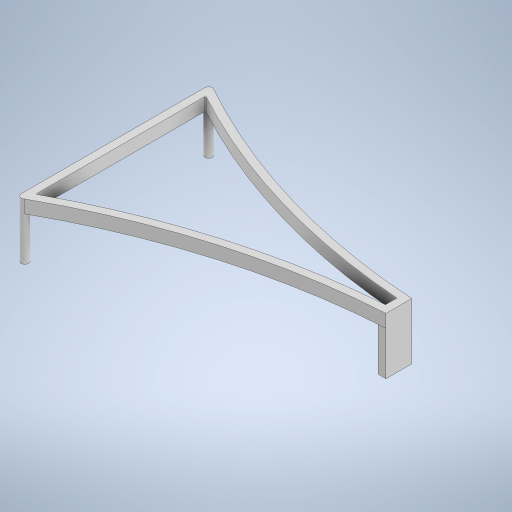
# Autodesk Inventor part: drzak_baterie
Saved by Autodesk Inventor 2024 (Build 280153000, 153)
## iProperties
Created: 2024-04-17
Part Number: drzak_baterie
Material: Všeobecné
Document SubType Name: Modeling
Designer: eliasla
Density: 1 g/cm^3
Appearance: Výchozí
Author: eliasla
Autodesk Inventor part; units mm, degrees
ref_plane "YZ Plane" through (0, 0, 0) normal (1, 0, 0) x (0, 1, 0)
ref_plane "XZ Plane" through (0, 0, 0) normal (0, 1, 0) x (-1, 0, 0)
ref_plane "XY Plane" through (0, 0, 0) normal (0, 0, 1) x (1, 0, 0)
sketch "Náčrt1" plane through (0, 0, 0) normal (0, 0, 1) x (1, 0, 0)
  line L0 (47.8317, -5) -> (50.8317, -5)
  line L1 (50.8317, -5) -> (50.8317, 5)
  line L2 (50.8317, 5) -> (47.8317, 5)
  line L3 (47.8317, 5) -> (47.8317, -5)
  line L4 (47.8317, -5) -> (50.8317, 5) construction
  line L5 (50.8317, -5) -> (47.8317, 5) construction
  circle A0 centre (-58.7223, 35.7005) radius 1.45
  circle A1 centre (-58.7223, -35.5995) radius 1.45
  point P0 (0, 0)
  point P1 (50.8317, 0)
  point P2 (-60.1683, 0.0505)
  dimension "d7" = 10
  dimension "d8" = 5
  dimension "d13" = 2.9
  dimension "d14" = 74.2
  constraints: 12 end point, 2 centre point, 2 parallel, 1 horizontal, 1 midpoint, 1 perpendicular
  measures "d7" distance of L0.end L1.end
  measures "d8" vertical distance of point (0, 0) L2.end
  measures "d13" diameter of A0
extrude "Vysunutí1" add sketch "Náčrt1" along normal blind 17
sketch "Náčrt2" plane through (-58.7223, 35.7005, 17) normal (0, 0, 1) x (1, 0, 0)
  circle A0 centre (0, 0) radius 1.45 projected
  line L0 (109.5541, -40.7005) -> (109.5541, -30.7005) projected
  arc A1 (0.9632, 1.0839) -> (109.5541, -30.7005) centre (125.5077, 225.1962) ccw
  circle A2 centre (0, -71.3) radius 1.45 projected
  line L1 (-1.45, 0) -> (-1.45, -71.3)
  arc A3 (109.5541, -40.7005) -> (0.9632, -72.3839) centre (125.3027, -296.61) ccw
  arc A4 (1.55, -3.0822) -> (1.9226, -2.8646) centre (0, 0) ccw
  line L2 (106.5541, -33.504) -> (106.5541, -37.8971)
  arc A5 (106.5541, -37.8971) -> (1.8423, -68.4842) centre (125.3027, -296.61) ccw
  arc A6 (1.8423, -68.4842) -> (1.55, -68.3189) centre (0, -71.4011) ccw
  line L3 (106.5541, -37.8971) -> (106.5541, -33.504)
  line L4 (1.55, -3.0822) -> (1.55, -68.3189)
  arc A7 (1.9226, -2.8646) -> (106.5541, -33.504) centre (125.5077, 225.1962) ccw
  line L5 (109.5541, -30.7005) -> (109.5541, -40.7005)
  arc A8 (0.4127, -72.69) -> (0.9632, -72.3839) centre (0, -71.3) ccw
  arc A9 (0.9632, 1.0839) -> (-1.45, 0) centre (0, 0) ccw
  arc A10 (0.9632, 1.0839) -> (-1.45, 0) centre (0, 0) ccw
  arc A11 (-1.45, -71.3) -> (0.9632, -72.3839) centre (0, -71.3) ccw
  point P0 (58.7223, -35.7005)
  point P1 (3.4391, -0.2742)
  point P2 (-1.45, -3.1305)
  point P3 (3.4391, -71.1268)
  point P4 (-1.45, -68.2706)
  point P5 (109.5541, -35.7005)
  point P6 (106.5541, -35.7005)
  dimension "d20" = 2
  dimension "d23" = 3
  constraints: 26 point on circle, 10 centre point, 10 end point, 4 coincident, 2 collinear, 2 midpoint, 1 parallel, 1 point on line, 1 tangent, 1 vertical
  measures "d20" radial gap between concentric circles of A4 A0
  measures "d23" distance of point (109.554, -35.701) point (106.554, -35.701)
extrude "Vysunutí2" add sketch "Náčrt2" along normal blind 5
